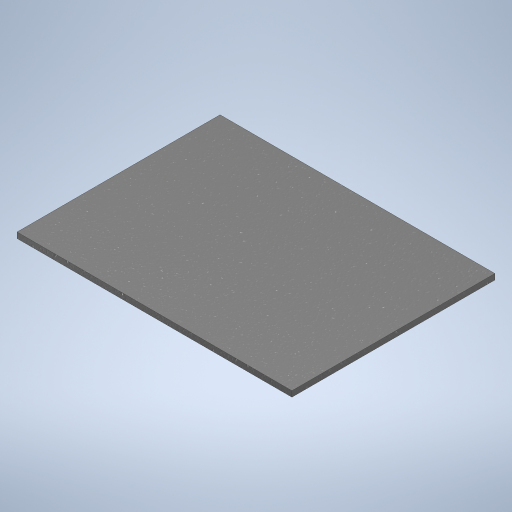
# Autodesk Inventor part: BottomHalfofSides_Ocampo
Saved by Autodesk Inventor 2023 (Build 270158000, 158)
## iProperties
Created: 2025-03-05
Part Number: BottomHalfofSides_Ocampo
Material: Generic
Document SubType Name: Modeling
Designer: FrameUser
Density: 1 g/cm^3
Appearance: Default
Author: FrameUser
Autodesk Inventor part; units mm, degrees
ref_plane "YZ Plane" through (0, 0, 0) normal (1, 0, 0) x (0, 1, 0)
ref_plane "XZ Plane" through (0, 0, 0) normal (0, 1, 0) x (-1, 0, 0)
ref_plane "XY Plane" through (0, 0, 0) normal (0, 0, 1) x (1, 0, 0)
sketch "Sketch1" plane through (0, 0, 0) normal (0, 1, 0) x (-1, 0, 0)
  line L0 (0, 0) -> (-309.5625, 0)
  line L1 (-309.5625, 0) -> (-309.5625, -228.6)
  line L2 (-309.5625, -228.6) -> (0, -228.6)
  line L3 (0, -228.6) -> (0, 0)
  dimension "d0" = 309.5625
  dimension "d1" = 228.6
  dimension "d2" = 309.5625
  constraints: 8 end point, 2 horizontal, 1 perpendicular
  measures "d0" distance of L0.start L0.end
  measures "d1" distance of L0.end L1.end
  measures "d2" distance of L1.end L2.end
extrude "Extrusion1" add sketch "Sketch1" along normal blind 6.35
body "Solid1"
